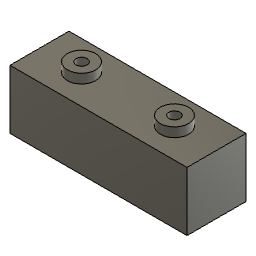
Battery Block (Autodesk Fusion 360 design; units mm, degrees)
Autodesk Fusion 360 part; units mm, degrees
sketch "Sketch1" plane through (0, 0, 0) normal (0, 1, 0) x (1, 0, 0)
  line L0 (0, 0) -> (76.2, 0)
  line L1 (76.2, 0) -> (76.2, 25.4)
  line L2 (76.2, 25.4) -> (0, 25.4)
  line L3 (0, 25.4) -> (0, 0)
  dimension "d1" = 76.2
  dimension "d2" = 25.4
  constraint horizontal L0
  constraint vertical L1
  constraint horizontal L2
  constraint vertical L3
  constraint coincident L0.start L3.end
  measures "d1" distance of L0.start L0.end
  measures "d2" distance of L0.start L2.end
extrude "Extrude1" add sketch "Sketch1" along normal blind 25.4
sketch "Sketch2" plane through (0, 25.4, 0) normal (0, 1, 0) x (-1, 0, 0)
  line L0 (0, -25.4) -> (0, 0)
  line L1 (0, 0) -> (-76.2, 0)
  line L2 (-76.2, 0) -> (-76.2, -25.4)
  line L3 (-76.2, -25.4) -> (0, -25.4)
  circle A0 centre (-18.1, -12.7) radius 6.096
  circle A1 centre (-58.1, -12.7) radius 6.096
  dimension "d6" = 12.192
  dimension "d8" = 12.192
  measures "d6" diameter of A0
  measures "d8" diameter of A1
extrude "Extrude2" add sketch "Sketch2" along normal blind 4 contours A0 | A1
sketch "Sketch3" plane through (0, 29.4, 0) normal (0, 1, 0) x (-1, 0, 0)
  circle A0 centre (-18.1, -12.7) radius 6.096
  circle A1 centre (-18.1, -12.7) radius 2.3813
  dimension "d11" = 4.7625
  constraint concentric A0 A1
  measures "d11" diameter of A1
extrude "Extrude3" cut sketch "Sketch3" against normal blind 12.7 contours A1
sketch "Sketch4" plane through (0, 29.4, 0) normal (0, 1, 0) x (-1, 0, 0)
  circle A0 centre (-58.1, -12.7) radius 6.096
  circle A1 centre (-58.1, -12.7) radius 2.3813
  dimension "d14" = 4.7625
  constraint concentric A0 A1
  measures "d14" diameter of A1
extrude "Extrude4" cut sketch "Sketch4" against normal blind 12.7 contours A1
